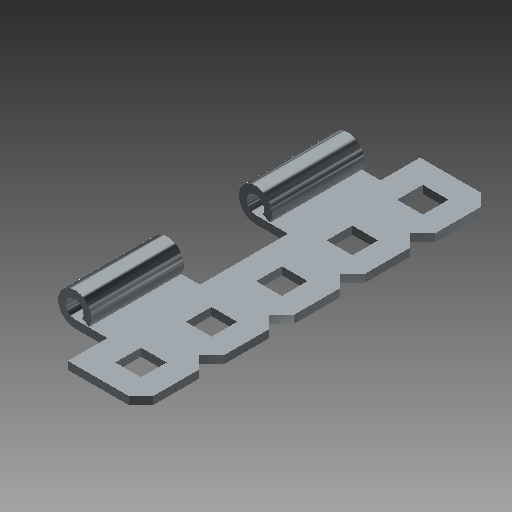
# Autodesk Inventor part: 275-1272
Saved by Autodesk Inventor 2018 (Build 220112000, 112)
## iProperties
Category: Structure
Company: Autodesk Inc.
Created: 2012-02-08
Part Number: 275-1272
Document SubType Name: Modeling
Designer: Autodesk Inc.
Density: 1 g/cm^3
Catalog Web Link: http://www.vexrobotics.com/products/accessories/structure/275-1272.html
Vendor: VEX
Material: Generic
Appearance: Zinc
Author: Autodesk Inc.
Autodesk Inventor part; units mm, degrees
ref_plane "YZ Plane" through (0, 0, 0) normal (1, 0, 0) x (0, 1, 0)
ref_plane "XZ Plane" through (0, 0, 0) normal (0, 1, 0) x (-1, 0, 0)
ref_plane "XY Plane" through (0, 0, 0) normal (0, 0, 1) x (1, 0, 0)
sketch "Sketch1" plane through (0, 0, 0) normal (0, 0, 1) x (1, 0, 0)
  line L0 (2.5847, -1.4923) -> (1.3748, -0.7938)
  arc A0 (2.5847, -1.4923) -> (0, -2.9845) centre (0, 0) ccw
  arc A1 (1.3748, -0.7938) -> (0, -1.5875) centre (0, 0) ccw
  arc A2 (1.3748, -0.7938) -> (0, -1.5875) centre (0, 0) ccw
  line L1 (0, -1.5875) -> (16.8049, -1.5875)
  line L2 (16.8049, -2.9845) -> (0, -2.9845)
  arc A3 (2.5847, -1.4923) -> (0, -2.9845) centre (0, 0) ccw
  line L3 (2.5847, -1.4923) -> (1.3748, -0.7938)
  line L4 (19.05, -1.5875) -> (16.8049, -1.5875)
  line L5 (19.05, -2.9845) -> (16.8049, -2.9845)
  line L6 (19.05, -1.5875) -> (19.05, -2.9845)
  point P0 (0, 0)
  point P1 (15.875, -2.9845)
  constraints: 14 end point, 8 point on circle, 4 centre point
extrude "Extrusion1" add sketch "Sketch1" against normal blind 63.5
sketch "Sketch2" plane through (0, -2.9845, 0) normal (0, -1, 0) x (1, 0, 0)
  line L0 (19.05, -23.1549) -> (19.05, -14.9451)
  line L1 (19.05, -14.9451) -> (16.8049, -12.7)
  line L2 (16.8049, -12.7) -> (19.05, -10.4549)
  line L3 (19.05, -10.4549) -> (19.05, -2.2451)
  line L4 (19.05, -2.2451) -> (16.8049, 0)
  line L5 (-2.9845, 0) -> (16.8049, 0)
  line L6 (0, -7.1247) -> (0, 0)
  line L7 (5.8525, -7.1247) -> (-2.9845, -7.1247)
  line L8 (5.8525, -39.6875) -> (5.8525, 0)
  line L9 (5.8525, -23.8125) -> (-2.9845, -23.8125)
  line L10 (0, -39.6875) -> (0, -23.8125)
  line L11 (5.8525, -39.6875) -> (-2.9845, -39.6875)
  line L12 (5.8525, -63.5) -> (5.8525, -39.6875)
  line L13 (-2.9845, -56.3753) -> (5.8525, -56.3753)
  line L14 (0, -63.5) -> (0, -56.3753)
  line L15 (16.8049, -63.5) -> (-2.9845, -63.5)
  line L16 (16.8049, -63.5) -> (19.05, -61.2549)
  line L17 (19.05, -61.2549) -> (19.05, -53.0451)
  line L18 (19.05, -53.0451) -> (16.8049, -50.8)
  line L19 (16.8049, -50.8) -> (19.05, -48.5549)
  line L20 (19.05, -48.5549) -> (19.05, -40.3451)
  line L21 (19.05, -40.3451) -> (16.8049, -38.1)
  line L22 (16.8049, -38.1) -> (19.05, -35.8549)
  line L23 (19.05, -35.8549) -> (19.05, -27.6451)
  line L24 (19.05, -27.6451) -> (16.8049, -25.4)
  line L25 (16.8049, -25.4) -> (19.05, -23.1549)
  line L26 (15.0114, -42.1386) -> (15.0114, -46.7614)
  line L27 (15.0114, -46.7614) -> (10.3886, -46.7614)
  line L28 (10.3886, -46.7614) -> (10.3886, -42.1386)
  line L29 (10.3886, -42.1386) -> (15.0114, -42.1386)
  line L30 (15.0114, -29.4386) -> (15.0114, -34.0614)
  line L31 (15.0114, -34.0614) -> (10.3886, -34.0614)
  line L32 (10.3886, -34.0614) -> (10.3886, -29.4386)
  line L33 (10.3886, -29.4386) -> (15.0114, -29.4386)
  line L34 (15.0114, -16.7386) -> (15.0114, -21.3614)
  line L35 (15.0114, -21.3614) -> (10.3886, -21.3614)
  line L36 (10.3886, -21.3614) -> (10.3886, -16.7386)
  line L37 (10.3886, -16.7386) -> (15.0114, -16.7386)
  line L38 (15.0114, -4.0386) -> (15.0114, -8.6614)
  line L39 (15.0114, -8.6614) -> (10.3886, -8.6614)
  line L40 (10.3886, -8.6614) -> (10.3886, -4.0386)
  line L41 (10.3886, -4.0386) -> (15.0114, -4.0386)
  line L42 (15.0114, -54.8386) -> (15.0114, -59.4614)
  line L43 (15.0114, -59.4614) -> (10.3886, -59.4614)
  line L44 (10.3886, -59.4614) -> (10.3886, -54.8386)
  line L45 (10.3886, -54.8386) -> (15.0114, -54.8386)
  line L46 (-2.9845, 0) -> (-2.9845, -63.5) projected
  line L47 (19.05, -53.0451) -> (19.05, -48.5549)
  line L48 (19.05, -40.3451) -> (19.05, -35.8549)
  line L49 (19.05, -27.6451) -> (19.05, -23.1549)
  line L50 (19.05, -14.9451) -> (19.05, -10.4549)
  line L51 (0, 0) -> (16.8049, 0) projected
  line L52 (16.8049, -63.5) -> (19.05, -63.5)
  line L53 (19.05, -63.5) -> (19.05, -61.2549)
  line L54 (19.05, -2.2451) -> (19.05, 0)
  line L55 (19.05, 0) -> (16.8049, 0)
  line L56 (16.8049, -63.5) -> (19.05, -61.2549)
  line L57 (19.05, -2.2451) -> (16.8049, 0)
  line L58 (0, -63.5) -> (16.8049, -63.5) projected
  line L59 (5.8525, -7.1247) -> (-2.9845, -7.1247)
  line L60 (-2.9845, -7.1247) -> (-2.9845, 0)
  line L61 (-2.9845, 0) -> (5.8525, 0)
  line L62 (5.8525, 0) -> (5.8525, -7.1247)
  point P0 (15.875, -31.75)
  constraints: 120 end point, 19 point on line, 5 collinear, 3 parallel, 3 perpendicular, 1 horizontal
extrude "Extrusion2" cut sketch "Sketch2" against normal blind 6.35 contours L49 L24 L25 | L1 L2 L50 | L48 L21 L22 | L4 L55 L54 | L47 L18 L19 | L8 L7 L6 L5 | L6 L7 L46 L5 | L53 L52 L16 | L8 L11 L10 L9 | L10 L11 L46 L9 | L15 L14 L13 L12 | L15 L46 L13 L14 | L26 L27 L28 L29 | L30 L31 L32 L33 | L34 L35 L36 L37 | L38 L39 L40 L41 | L42 L43 L44 L45
sketch "Sketch3" plane through (0, -2.9845, 0) normal (0, -1, 0) x (1, 0, 0)
  line L0 (15.0114, -8.6614) -> (10.3886, -8.6614) projected
  circle A0 centre (12.7, -6.35) radius 2.3114
  constraints: 1 centre point, 1 tangent
surface extrude "ExtrusionSrf1" sketch "Sketch3" against normal up to surface (1.397 mm away) shown no curves A0
pattern_linear "Rectangular Pattern1" count 5 spacing 12.7 along (0, 0, -1) of "ExtrusionSrf1"
body "Solid1"
body "Srf1"
body "Srf2"
body "Srf3"
body "Srf4"
body "Srf5"
